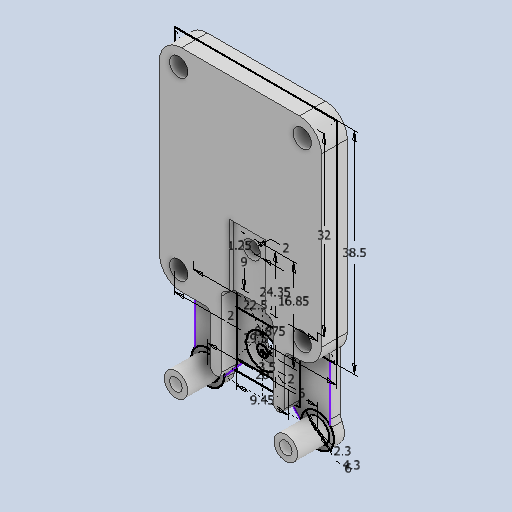
# Autodesk Inventor part: Crossbow CNC VC4_T1_Assy_simplified_V2
Saved by Autodesk Inventor 2024 (Build 280153000, 153)
## iProperties
Created: 2026-03-13
Part Number: Crossbow CNC VC4_T1_Assy_simplified_V2
Material: Generic
Document SubType Name: Modeling
Designer: RidDleZ
Density: 1 g/cm^3
Appearance: Default
Author: RidDleZ
## iProperties of the stored document Crossbow CNC VC4_T1_Assy_simplified_V2_3DPrint.ipt
Created: 2026-03-14
Part Number: Crossbow CNC VC4_T1_Assy_simplified_V2_3DPrint
Material: Generic
Document SubType Name: Modeling
Designer: RidDleZ
Density: 1 g/cm^3
Appearance: Default
Author: RidDleZ
Autodesk Inventor part; units mm, degrees
ref_plane "YZ Plane" through (0, 0, 0) normal (1, 0, 0) x (0, 1, 0)
ref_plane "XZ Plane" through (0, 0, 0) normal (0, 1, 0) x (-1, 0, 0)
ref_plane "XY Plane" through (0, 0, 0) normal (0, 0, 1) x (1, 0, 0)
sketch "Sketch1" plane through (0, 0, 0) normal (0, 0, 1) x (1, 0, 0)
  line L0 (-11.25, 16) -> (11.25, 16) construction
  line L1 (11.25, 16) -> (11.25, -16) construction
  line L2 (11.25, -16) -> (-11.25, -16) construction
  line L3 (-11.25, -16) -> (-11.25, 16) construction
  line L4 (0, 16) -> (0, -16) construction
  line L5 (-14.75, 19.25) -> (14.75, 19.25)
  line L6 (14.75, 19.25) -> (14.75, -19.25)
  line L7 (14.75, -19.25) -> (-14.75, -19.25)
  line L8 (-14.75, -19.25) -> (-14.75, 19.25)
  line L9 (-14.75, 19.25) -> (14.75, -19.25) construction
  line L10 (14.75, 19.25) -> (-14.75, -19.25) construction
  line L11 (1.25, -16) -> (1.25, -7) construction
  line L12 (-8.75, -31.35) -> (11.25, -31.35) construction
  circle A0 centre (11.25, -31.35) radius 3
  circle A1 centre (-8.75, -31.35) radius 3
  line L13 (1.25, -31.35) -> (1.25, -7) construction
  circle A2 centre (1.25, -23.85) radius 3
  circle A3 centre (1.25, -23.85) radius 1
  circle A4 centre (1.25, -7) radius 1
  line L14 (-3.475, -14.975) -> (5.975, -14.975)
  line L15 (5.975, -14.975) -> (5.975, -27.35)
  line L16 (5.975, -27.35) -> (-3.475, -27.35)
  line L17 (-3.475, -27.35) -> (-3.475, -14.975)
  line L18 (-3.475, -14.975) -> (5.975, -27.35) construction
  line L19 (5.975, -14.975) -> (-3.475, -27.35) construction
  circle A5 centre (11.25, -31.35) radius 2.15
  circle A6 centre (-8.75, -31.35) radius 2.15
  line L20 (13.5, -29.3657) -> (13.5, -19.25)
  line L21 (-11, -29.3657) -> (-11, -19.25)
  line L22 (-5.75, -31.35) -> (-2.2423, -27.35)
  line L23 (-2.2423, -27.35) -> (4.7423, -27.35)
  line L24 (4.7423, -27.35) -> (8.25, -31.35)
  line L25 (-5.475, -12.975) -> (7.975, -12.975)
  line L26 (7.975, -12.975) -> (7.975, -29.35)
  line L27 (7.975, -29.35) -> (-5.475, -29.35)
  line L28 (-5.475, -29.35) -> (-5.475, -12.975)
  line L29 (-3.475, -27.35) -> (-3.475, -29.35)
  line L30 (5.975, -27.35) -> (5.975, -29.35)
  circle A7 centre (11.25, -31.35) radius 1.15
  circle A8 centre (-8.75, -31.35) radius 1.15
  point P0 (0, 0)
  point P1 (1.25, -21.1625)
  point P2 (0, 0)
  point P3 (0, 0)
  point P4 (1.25, -27.35)
  point P5 (-5.475, -19.25)
  point P6 (7.975, -19.25)
  dimension "d0" = 22.5
  dimension "d1" = 32
  dimension "d2" = 29.5
  dimension "d3" = 38.5
  dimension "d4" = 9
  dimension "d5" = 1.25
  dimension "d7" = 20
  dimension "d8" = 6
  dimension "d11" = 24.35
  dimension "d12" = 6
  dimension "d13" = 16.85
  dimension "d14" = 2
  dimension "d15" = 2
  dimension "d16" = 9.45
  dimension "d18" = 8.875
  dimension "d19" = 4.3
  dimension "d20" = 3.5
  dimension "d23" = 2
  dimension "d48" = 2.3
  constraints: 62 end point, 14 coincident, 10 midpoint, 10 point on line, 9 centre point, 9 perpendicular, 8 parallel, 5 horizontal, 4 point on circle, 3 equal radius, 1 vertical, 3 other
  measures "d0" distance of L1.end L2.end
  measures "d1" distance of L0.end L1.end
  measures "d2" distance of L6.end L7.end
  measures "d3" distance of L5.end L6.end
  measures "d4" distance of L11.start L11.end
  measures "d5" distance between parallel lines of L4 L11
  measures "d7" distance of L12.start L12.end
  measures "d8" diameter of A0
  measures "d11" distance of L11.end L13.start
  measures "d12" diameter of A2
  measures "d13" distance of L11.end A2.centre
  measures "d14" diameter of A3
  measures "d15" diameter of A4
  measures "d16" distance of L15.end L16.end
  measures "d18" distance from line of A2.centre L14
  measures "d19" diameter of A5
  measures "d20" distance from line of A2.centre L23
  measures "d23" distance between parallel lines of L17 L28
  measures "d48" diameter of A7
extrude "Extrusion1" add sketch "Sketch1" against normal blind 2 contours L5 L6 L7 L26 L25 L28 L8 | L7 L28 L27 L22 A1 L21 | L20 A0 L24 L27 L26 L7 | L28 L25 L26 L7 L15 L14 L17 | L7 L17 L29 L22 L27 L28 | A1 | L26 L27 L24 L30 L15 L7 | A0 | L17 L14 L15 L7 | L7 L15 L16 L17 | L16 L22 L29 | L30 L24 L16 | A2 | A5 | A6 | A7 | A8
extrude "Extrusion2" add sketch "Sketch1" along normal blind 2.7 contours L5 L6 L7 L26 L25 L28 L8 | L28 L25 L26 L7 L15 L14 L17 | L7 L17 L29 L22 L27 L28 | L26 L27 L24 L30 L15 L7 | L22 L29 L27 | L27 L30 L24
fillet "Fillet1" radius 1 6 edges at (7.975, -29.35, 1.35) (5.975, -29.35, 1.35) (-3.475, -29.35, 1.35) (-5.475, -29.35, 1.35) (7.975, -19.25, 1.35) (-5.475, -19.25, 1.35)
fillet "Fillet2" radius 1.325 2 edges at (-3.475, -14.975, 1.35) (5.975, -14.975, 1.35)
extrude "Extrusion3" cut sketch "Sketch1" against normal blind 1.6 contours A2
hole "mnt_holes" at (-11.25, 16, 0) at (11.25, 16, 0) at (11.25, -16, 0) at (-11.25, -16, 0) direction (0, 0, -1) diameter 3.35 end through all both
sketch "Sketch2" plane through (0, 0, 2.7) normal (0, 0, 1) x (1, 0, 0)
  line L0 (-2, -3.4) -> (4.5, -3.4)
  line L1 (4.5, -3.4) -> (4.5, -14.975)
  line L2 (4.5, -14.975) -> (-2, -14.975)
  line L3 (-2, -14.975) -> (-2, -3.4)
  line L4 (-2, -3.4) -> (4.5, -14.975) construction
  line L5 (4.5, -3.4) -> (-2, -14.975) construction
  line L6 (1.25, -3.4) -> (1.25, -7) construction
  line L7 (-2.15, -14.975) -> (4.65, -14.975) construction
  line L8 (4.65, -14.975) -> (-2.15, -14.975) construction
  point P0 (0, 0)
  point P1 (1.25, -9.1875)
  point P2 (1.25, -14.975)
  dimension "d40" = 6.5
  dimension "d42" = 3.6
  constraints: 14 end point, 5 midpoint, 2 parallel, 1 coincident, 1 horizontal, 1 perpendicular, 1 vertical
  measures "d40" distance of L1.end L2.end
  measures "d42" distance of L6.start L6.end
extrude "Extrusion4" cut sketch "Sketch2" against normal blind 0.8
chamfer "Chamfer2" distance 0.6 angle 45 1 edges at (0.25, -7, 1.9)
extrude "Extrusion5" add sketch "Sketch1" along normal blind 5.7 contours A5 | A6
fillet "Fillet3" radius 4 4 edges at (14.75, -19.25, 0.35) (-14.75, -19.25, 0.35) (-14.75, 19.25, 0.35) (14.75, 19.25, 0.35)
fillet "Fillet4" radius 2 6 edges at (-2.2423, -27.35, -1) (4.7423, -27.35, -1) (-5.75, -31.35, -1) (8.25, -31.35, -1) (-11, -29.3657, -1) (13.5, -29.3657, -1)
sketch "Sketch3" plane through (0, 0, -2) normal (0, 0, -1) x (-1, 0, 0)
  circle A0 centre (-1.25, -7) radius 1 projected
  circle A1 centre (-1.25, -7) radius 2.1
  point P0 (0, 0)
  dimension "d53" = 4.2
  constraints: 1 centre point, 1 coincident
  measures "d53" diameter of A1
extrude "Extrusion6" cut sketch "Sketch3" against normal blind 1.7
